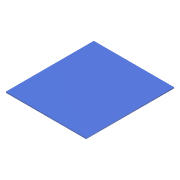
# Autodesk Inventor part: AcrylicDiagonal
Saved by Autodesk Inventor 2014 (Build 180170000, 170)
## iProperties
Created: 2014-08-11
Part Number: AcrylicDiagonal
Material: Generic
Document SubType Name: Modeling
Designer: Peele
Density: 1 g/cm^3
Appearance: Clear - Blue
Author: Peele
Autodesk Inventor part; units mm, degrees
ref_plane "YZ Plane" through (0, 0, 0) normal (1, 0, 0) x (0, 1, 0)
ref_plane "XZ Plane" through (0, 0, 0) normal (0, 1, 0) x (-1, 0, 0)
ref_plane "XY Plane" through (0, 0, 0) normal (0, 0, 1) x (1, 0, 0)
sketch "Sketch1" plane through (0, 0, 0) normal (0, 0, 1) x (1, 0, 0)
  line L0 (-105, -115) -> (105, -115)
  line L1 (105, -115) -> (105, 115)
  line L2 (105, 115) -> (-105, 115)
  line L3 (-105, 115) -> (-105, -115)
  line L4 (-105, -115) -> (105, 115) construction
  line L5 (105, -115) -> (-105, 115) construction
  point P0 (0, 0)
  dimension "d0" = 230
  dimension "d1" = 210
  constraints: 12 end point, 2 midpoint, 2 parallel, 1 horizontal, 1 perpendicular
  measures "d0" distance of L2.end L0.start
  measures "d1" distance of L0.start L0.end
extrude "Extrusion1" add sketch "Sketch1" along normal blind 3
body "Solid1"
